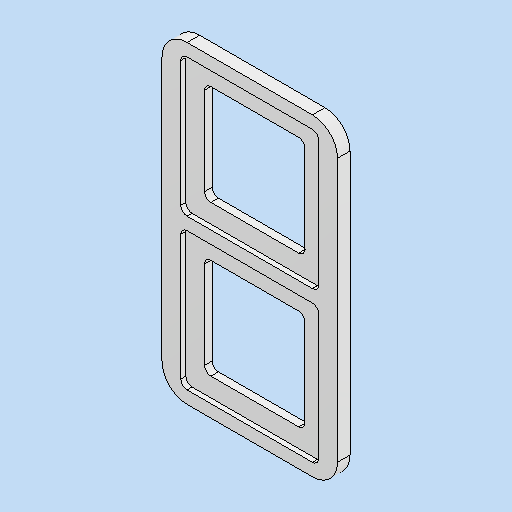
# Autodesk Inventor part: SampleTray
Saved by Autodesk Inventor 2025 (Build 290162000, 162)
## iProperties
Created: 2024-08-28
Part Number: SampleTray
Material: UHMW, White
Document SubType Name: Modeling
Designer: kuzmin
Density: 0.94 g/cm^3
Appearance: Smooth - White
Author: kuzmin
Autodesk Inventor part; units mm, degrees
ref_plane "YZ Plane" through (0, 0, 0) normal (1, 0, 0) x (0, 1, 0)
ref_plane "XZ Plane" through (0, 0, 0) normal (0, 1, 0) x (-1, 0, 0)
ref_plane "XY Plane" through (0, 0, 0) normal (0, 0, 1) x (1, 0, 0)
sketch "Sketch1" plane through (0, 0, 0) normal (0, 0, 1) x (1, 0, 0)
  line L0 (-7, 12.5) -> (7, 12.5)
  line L1 (7, 12.5) -> (7, -12.5)
  line L2 (7, -12.5) -> (-7, -12.5)
  line L3 (-7, -12.5) -> (-7, 12.5)
  point P0 (0, 0)
  point P1 (7, 0)
  point P2 (0, 12.5)
  dimension "d0" = 14
  dimension "d1" = 25
  constraints: 8 end point, 2 midpoint, 2 parallel, 1 horizontal, 1 horizontal alignment, 1 perpendicular, 1 vertical alignment
  measures "d0" distance of L0.start L0.end
  measures "d1" distance of L0.end L1.end
extrude "Extrusion1" add sketch "Sketch1" along normal blind 1
sketch "Sketch2" plane through (0, 0, 1) normal (0, 0, 1) x (1, 0, 0)
  line L0 (-5.5, 11.5) -> (5.5, 11.5)
  line L1 (5.5, 11.5) -> (5.5, 0.5)
  line L2 (5.5, 0.5) -> (-5.5, 0.5)
  line L3 (-5.5, 0.5) -> (-5.5, 11.5)
  line L4 (7, 12.5) -> (-7, 12.5) projected
  point P0 (0, 0)
  point P1 (0, 11.5)
  dimension "d4" = 11
  dimension "d5" = 11
  dimension "d6" = 1
  constraints: 8 end point, 2 parallel, 1 horizontal, 1 midpoint, 1 perpendicular, 1 vertical alignment
  measures "d4" distance of L0.start L0.end
  measures "d5" distance of L0.end L1.end
  measures "d6" distance between parallel lines of L4 L0
extrude "Extrusion2" cut sketch "Sketch2" against normal blind 0.4
sketch "Sketch3" plane through (0, 0, 0.6) normal (0, 0, 1) x (1, 0, 0)
  line L0 (5.5, 0.5) -> (-5.5, 0.5) projected
  line L1 (5.5, 11.5) -> (5.5, 0.5) projected
  line L2 (-5.5, 11.5) -> (5.5, 11.5) projected
  line L3 (-5.5, 0.5) -> (-5.5, 11.5) projected
  line L4 (4, 10) -> (4, 2)
  line L5 (4, 2) -> (-4, 2)
  line L6 (-4, 2) -> (-4, 10)
  line L7 (-4, 10) -> (4, 10)
  point P0 (0, 0)
  dimension "d9" = 1.5
  constraints: 8 end point, 3 other
  measures "d9" distance between parallel lines of L2 L7
extrude "Extrusion3" cut sketch "Sketch3" against normal through all contours L4 L5 L6 L7
mirror "Mirror1" about plane through (0, 0, 0) normal (0, 1, 0) of "Extrusion3", "Extrusion2"
fillet "Fillet1" radius 2 4 edges at (7, 12.5, 0.5) (7, -12.5, 0.5) (-7, -12.5, 0.5) (-7, 12.5, 0.5)
fillet "Fillet2" radius 0.5 8 edges at (-4, 2, 0.3) (-4, 10, 0.3) (4, 10, 0.3) (4, 2, 0.3) (4, -2, 0.3) (-4, -2, 0.3) (-4, -10, 0.3) (4, -10, 0.3)
fillet "Fillet3" radius 0.5 8 edges at (-5.5, 11.5, 0.8) (5.5, 11.5, 0.8) (5.5, 0.5, 0.8) (-5.5, 0.5, 0.8) (-5.5, -0.5, 0.8) (5.5, -0.5, 0.8) (5.5, -11.5, 0.8) (-5.5, -11.5, 0.8)
body "Solid1"
